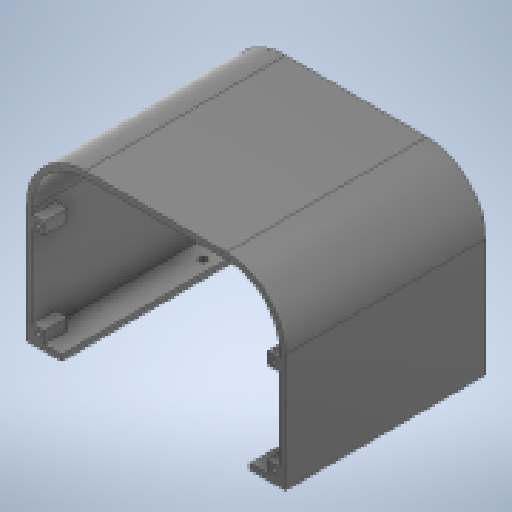
# Autodesk Inventor part: speaker
Saved by Autodesk Inventor 2026.2 (Build 302298010, 298A)
## iProperties
Created: 2026-05-26
Part Number: speaker
Material: ABS Plastic
Document SubType Name: Modeling
Designer: chris
Density: 1.06 g/cm^3
Appearance: Smooth - White
Author: chris
Autodesk Inventor part; units mm, degrees
ref_plane "YZ Plane" through (0, 0, 0) normal (1, 0, 0) x (0, 1, 0)
ref_plane "XY Plane" through (0, 0, 0) normal (0, 0, 1) x (1, 0, 0)
sketch "Sketch1" plane through (0, 0, 0) normal (0, 1, 0) x (-1, 0, 0)
  line L0 (110, 85) -> (-110, 85)
  line L1 (-110, 85) -> (-110, -85)
  line L2 (-110, -85) -> (110, -85)
  line L3 (110, -85) -> (110, 85)
  line L4 (110, 85) -> (-110, -85) construction
  line L5 (-110, 85) -> (110, -85) construction
  point P0 (0, 0)
  dimension "d0" = 220
  dimension "d1" = 170
  constraints: 12 end point, 2 midpoint, 2 parallel, 1 horizontal, 1 perpendicular
  measures "d0" distance of L2.end L1.end
  measures "d1" distance of L1.end L0.end
extrude "Extrusion1" add sketch "Sketch1" along normal blind 5
sketch "Sketch2" plane through (0, 5, 0) normal (0, 1, 0) x (1, 0, 0)
  line L0 (-110, -85) -> (-105, -85)
  line L1 (-105, -85) -> (-105, 85)
  line L2 (-105, 85) -> (-110, 85)
  line L3 (-110, 85) -> (-110, -85)
  line L4 (-110, -85) -> (-105, 85) construction
  line L5 (-105, -85) -> (-110, 85) construction
  line L6 (-110, 85) -> (-110, -85) projected
  point P0 (0, 0)
  point P1 (-107.5, 0)
  dimension "d4" = 5
  dimension "d5" = 170
  dimension "d6" = 0
  constraints: 12 end point, 2 midpoint, 2 parallel, 1 horizontal, 1 horizontal alignment, 1 perpendicular
  measures "d4" distance of L2.end L1.end
  measures "d5" distance of L1.end L0.end
  measures "d6" distance between parallel lines of L6 L3
extrude "Extrusion2" add sketch "Sketch2" along normal blind 95
mirror "Mirror1" about plane through (0, 0, 0) normal (1, 0, 0) of "Extrusion2"
ref_plane "Work Plane1" through (0, 145, 0) normal (0, 1, 0) x (-1, 0, 0)
sketch "Sketch3" plane through (0, 145, 0) normal (0, 1, 0) x (-1, 0, 0)
  line L0 (60, 85) -> (-60, 85)
  line L1 (-60, 85) -> (-60, -85)
  line L2 (-60, -85) -> (60, -85)
  line L3 (60, -85) -> (60, 85)
  line L4 (60, 85) -> (-60, -85) construction
  line L5 (-60, 85) -> (60, -85) construction
  point P0 (0, 0)
  dimension "d10" = 120
  dimension "d11" = 170
  constraints: 12 end point, 2 midpoint, 2 parallel, 1 horizontal, 1 perpendicular
  measures "d10" distance of L2.end L1.end
  measures "d11" distance of L1.end L0.end
extrude "Extrusion3" add sketch "Sketch3" along normal blind 5
sketch "Sketch4" plane through (0, 0, 0) normal (0, -1, 0) x (1, 0, 0)
  line L0 (-80, -100) -> (80, -100)
  line L1 (80, -100) -> (80, 100)
  line L2 (80, 100) -> (-80, 100)
  line L3 (-80, 100) -> (-80, -100)
  line L4 (-80, -100) -> (80, 100) construction
  line L5 (80, -100) -> (-80, 100) construction
  point P0 (0, 0)
  dimension "d14" = 160
  dimension "d15" = 200
  constraints: 12 end point, 2 midpoint, 2 parallel, 1 horizontal, 1 perpendicular
  measures "d14" distance of L2.end L1.end
  measures "d15" distance of L1.end L0.end
extrude "Extrusion4" cut sketch "Sketch4" against normal blind 5
sketch "Sketch5" plane through (0, 0, 0) normal (0, 0, 1) x (1, 0, 0)
  line L0 (-110, 100) -> (-105, 100) projected
  line L1 (-60, 145) -> (-60, 150) projected
  arc A0 (-60, 147.5) -> (-107.5, 100) centre (-60, 100) ccw
  point P0 (0, 0)
  constraints: 2 point on circle, 1 centre point
sketch "Sketch6" plane through (0, 100, 0) normal (0, 1, 0) x (1, 0, 0)
  line L0 (-110, 85) -> (-105, 85)
  line L1 (-105, 85) -> (-105, -85)
  line L2 (-105, -85) -> (-110, -85)
  line L3 (-110, -85) -> (-110, 85)
  line L4 (-105, 85) -> (-110, 85) projected
  line L5 (-110, -85) -> (-105, -85) projected
  line L6 (-105, -85) -> (-105, 85) projected
  line L7 (-110, 85) -> (-110, -85) projected
  point P0 (0, 0)
  constraints: 8 end point, 4 collinear, 2 parallel, 1 horizontal, 1 perpendicular
sweep "Sweep1" add profiles "Sketch6" path "Sketch5" path curves A0
mirror "Mirror2" about plane through (0, 0, 0) normal (1, 0, 0) of "Sweep1"
sketch "Sketch7" plane through (0, 0, 0) normal (0, -1, 0) x (1, 0, 0)
  circle A0 centre (-90, -45) radius 3.1
  circle A1 centre (90, -45) radius 3.1
  line L0 (-80, -85) -> (-80, 85) projected
  line L1 (-80, -85) -> (-110, -85) projected
  point P0 (0, 0)
  point P1 (-95, -85)
  dimension "d20" = 6.2
  dimension "d21" = 6.2
  dimension "d22" = 180
  dimension "d23" = 10
  dimension "d24" = 40
  constraints: 2 centre point, 1 horizontal alignment, 1 midpoint
  measures "d20" diameter of A0
  measures "d21" diameter of A1
  measures "d22" distance of A1.centre A0.centre
  measures "d23" distance from line of L0 A0.centre
  measures "d24" vertical distance of point (-95, -85) A0.centre
extrude "Extrusion5" cut sketch "Sketch7" against normal blind 5
sketch "Sketch8" plane through (-80, 0, -85) normal (0, 0, -1) x (-1, 0, 0)
  line L0 (-160, 0) -> (-160, 5) projected
  line L1 (-185, 5) -> (-160, 5) projected
  line L2 (-185, 5) -> (-185, 100) projected
  arc A0 (-140, 145) -> (-185, 100) centre (-140, 100) ccw projected
  line L3 (-140, 145) -> (-20, 145) projected
  arc A1 (25, 100) -> (-20, 145) centre (-20, 100) ccw projected
  line L4 (25, 5) -> (25, 100) projected
  line L5 (0, 5) -> (25, 5) projected
  line L6 (0, 5) -> (0, 0) projected
  line L7 (0, 0) -> (30, 0) projected
  line L8 (30, 0) -> (30, 100) projected
  arc A2 (30, 100) -> (-20, 150) centre (-20, 100) ccw projected
  line L9 (-140, 150) -> (-20, 150) projected
  arc A3 (-140, 150) -> (-190, 100) centre (-140, 100) ccw projected
  line L10 (-190, 0) -> (-190, 100) projected
  line L11 (-190, 0) -> (-160, 0) projected
  line L12 (-160, 0) -> (0, 0)
  point P0 (-80, 0)
  constraints: 2 end point, 1 horizontal
extrude "Extrusion6" add sketch "Sketch8" against normal blind 3 contours L0 L1 L2 A0 L3 A1 L4 L5 L6 L12
sketch "Sketch9" plane through (110, 0, -85) normal (0, 0, -1) x (-1, 0, 0)
  line L0 (70, 0) -> (150, 0)
  line L1 (150, 0) -> (150, 35)
  line L2 (150, 35) -> (70, 35)
  line L3 (70, 35) -> (70, 0)
  line L4 (70, 0) -> (150, 35) construction
  line L5 (150, 0) -> (70, 35) construction
  line L6 (0, 0) -> (220, 0) projected
  line L7 (110, -30) -> (110, 180) projected
  point P0 (110, 0)
  point P1 (110, 17.5)
  dimension "d29" = 80
  dimension "d30" = 35
  constraints: 12 end point, 2 midpoint, 2 parallel, 1 collinear, 1 horizontal, 1 perpendicular, 1 point on line
  measures "d29" distance of L1.end L2.end
  measures "d30" distance between parallel lines of L0 L2
extrude "Extrusion7" cut sketch "Sketch9" against normal blind 3
sketch "Sketch10" plane through (-110, 0, -85) normal (0, 0, -1) x (-1, 0, 0)
  line L0 (-110.5, 40) -> (-109.5, 40)
  line L1 (-108.5, 41) -> (-108.5, 129)
  line L2 (-109.5, 130) -> (-110.5, 130)
  line L3 (-111.5, 129) -> (-111.5, 41)
  line L4 (-111.5, 40) -> (-108.5, 130) construction
  line L5 (-108.5, 40) -> (-111.5, 130) construction
  line L6 (-110, -30) -> (-110, 180) projected
  line L7 (-70, 0) -> (0, 0) projected
  arc A0 (-111.5, 41) -> (-110.5, 40) centre (-110.5, 41) ccw
  arc A1 (-109.5, 40) -> (-108.5, 41) centre (-109.5, 41) ccw
  arc A2 (-110.5, 130) -> (-111.5, 129) centre (-110.5, 129) ccw
  arc A3 (-108.5, 129) -> (-109.5, 130) centre (-109.5, 129) ccw
  point P0 (-110, 0)
  point P1 (-110, 85)
  dimension "d33" = 3
  dimension "d34" = 90
  dimension "d35" = 40
  dimension "d41" = 1
  dimension "d42" = 1
  constraints: 12 end point, 9 point on line, 8 point on circle, 8 tangent, 4 centre point, 2 equal radius, 2 midpoint, 2 parallel, 1 horizontal, 1 perpendicular
  measures "d33" distance of L5.end L4.end
  measures "d34" distance of L4.end L5.start
  measures "d35" distance between parallel lines of L7 L0
  measures "d41" radius of A0
  measures "d42" radius of A1
extrude "Extrusion8" cut sketch "Sketch10" against normal blind 3
pattern_linear "Rectangular Pattern1" count 29 spacing 6 along (1, 0, 0) of "Extrusion8" first direction both ways yes
fillet "Fillet1" radius 10 2 edges at (-40, 35, -83.5) (40, 35, -83.5)
sketch "Sketch11" plane through (80, 0, 85) normal (0, 0, 1) x (1, 0, 0)
  line L0 (-175, 15) -> (-190, 15)
  line L1 (-190, 15) -> (-190, 0)
  line L2 (-190, 0) -> (-175, 0)
  line L3 (-175, 0) -> (-175, 15)
  line L4 (15, 15) -> (30, 15)
  line L5 (30, 15) -> (30, 0)
  line L6 (30, 0) -> (15, 0)
  line L7 (15, 0) -> (15, 15)
  line L8 (-190, 0) -> (-190, 100) projected
  line L9 (-190, 0) -> (-160, 0) projected
  line L10 (30, 0) -> (30, 100) projected
  line L11 (0, 0) -> (30, 0) projected
  line L12 (-190, 95) -> (-175, 95)
  line L13 (-175, 95) -> (-175, 85)
  line L14 (-175, 85) -> (-190, 85)
  line L15 (-190, 85) -> (-190, 95)
  line L16 (15, 95) -> (30, 95)
  line L17 (30, 95) -> (30, 85)
  line L18 (30, 85) -> (15, 85)
  line L19 (15, 85) -> (15, 95)
  point P0 (-80, 0)
  point P1 (22.5, 85)
  point P2 (30, 85)
  dimension "d45" = 15
  dimension "d46" = 15
  dimension "d47" = 15
  dimension "d48" = 15
  dimension "d51" = 15
  dimension "d52" = 10
  dimension "d53" = 15
  dimension "d54" = 10
  dimension "d55" = 70
  dimension "d56" = 70
  constraints: 30 end point, 7 parallel, 6 collinear, 4 horizontal, 4 perpendicular, 1 midpoint, 1 vertical, 3 other
  measures "d45" distance of L0.start L0.end
  measures "d46" distance of L0.end L1.end
  measures "d47" distance of L4.start L4.end
  measures "d48" distance of L4.end L5.end
  measures "d51" distance of L13.end L14.end
  measures "d52" distance of L12.end L13.end
  measures "d53" distance of L17.end L18.end
  measures "d54" distance of L16.end L17.end
  measures "d55" distance between parallel lines of L14 L0
  measures "d56" distance from line of point (22.5, 85) L4
extrude "Extrusion9" add sketch "Sketch11" against normal blind 20
sketch "Sketch12" plane through (80, 0, 85) normal (0, 0, 1) x (1, 0, 0)
  circle A0 centre (-180, 10) radius 2
  circle A1 centre (-180, 90) radius 2
  circle A2 centre (20, 90) radius 2
  circle A3 centre (20, 10) radius 2
  line L0 (-160, 0) -> (-160, 15) projected
  line L1 (-175, 15) -> (-185, 15) projected
  line L2 (-175, 95) -> (-185, 95) projected
  line L3 (0, 15) -> (0, 0) projected
  point P0 (-80, 0)
  point P1 (-185, 100)
  point P2 (15, 15)
  point P3 (0, 0)
  point P4 (-184.7214, 105)
  dimension "d57" = 4
  dimension "d58" = 4
  dimension "d59" = 4
  dimension "d60" = 4
  dimension "d61" = 20
  dimension "d62" = 5
  dimension "d63" = 5
  dimension "d64" = 20
  constraints: 4 centre point, 2 horizontal alignment, 2 vertical alignment, 1 other
  measures "d57" diameter of A0
  measures "d58" diameter of A1
  measures "d59" diameter of A2
  measures "d60" diameter of A3
  measures "d61" distance from line of L0 A0.centre
  measures "d62" distance from line of L1 A0.centre
  measures "d64" distance from line of L3 A3.centre
extrude "Extrusion10" cut sketch "Sketch12" against normal blind 20
body "Solid1"
